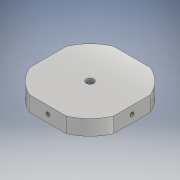
# Autodesk Inventor part: Bottom
Saved by Autodesk Inventor 2017 (Build 210142000, 142)
## iProperties
Created: 2016-06-22
Part Number: Bottom
Material: Generic
Document SubType Name: Modeling
Designer: Andres
Density: 1 g/cm^3
Appearance: Aluminum - Polished
Author: Andres
Autodesk Inventor part; units mm, degrees
ref_plane "YZ Plane" through (0, 0, 0) normal (1, 0, 0) x (0, 1, 0)
ref_plane "XZ Plane" through (0, 0, 0) normal (0, 1, 0) x (-1, 0, 0)
ref_plane "XY Plane" through (0, 0, 0) normal (0, 0, 1) x (1, 0, 0)
sketch "Sketch1" plane through (0, 0, 0) normal (0, 0, 1) x (1, 0, 0)
  circle A0 centre (0, 0) radius 30
  dimension "d0" = 60
  constraints: 1 centre point, 1 coincident
  measures "d0" diameter of A0
extrude "Extrusion1" add sketch "Sketch1" along normal blind 10
sketch "Sketch2" plane through (0, 0, 10) normal (0, 0, 1) x (1, 0, 0)
  line L0 (-27.5, -27.5) -> (27.5, -27.5)
  line L1 (27.5, -27.5) -> (27.5, 27.5)
  line L2 (27.5, 27.5) -> (-27.5, 27.5)
  line L3 (-27.5, 27.5) -> (-27.5, -27.5)
  line L4 (-27.5, -27.5) -> (27.5, 27.5) construction
  line L5 (27.5, -27.5) -> (-27.5, 27.5) construction
  point P0 (0, 0)
  dimension "d3" = 55
  dimension "d4" = 55
  constraints: 12 end point, 2 midpoint, 2 parallel, 1 horizontal, 1 perpendicular
  measures "d3" distance of L2.end L1.end
  measures "d4" distance of L1.end L0.end
extrude "Extrusion2" cut sketch "Sketch2" against normal blind 10 keep common part
sketch "Sketch3" plane through (-27.5, -11.9896, 10) normal (-1, 0, 0) x (0, 0, 1)
  point P0 (-10, 11.9896)
sketch "Sketch4" plane through (0, 0, 10) normal (0, 0, 1) x (1, 0, 0)
  circle A0 centre (0, 0) radius 2.5
  dimension "d7" = 5
  constraints: 1 centre point, 1 coincident
  measures "d7" diameter of A0
extrude "Extrusion3" cut sketch "Sketch4" against normal blind 10
sketch "Sketch9" plane through (-11.9896, -27.5, 10) normal (0, -1, 0) x (1, 0, 0)
  line L0 (23.9792, 0) -> (0, 0) projected
  point P0 (11.9896, -10)
  point P1 (11.9896, -5)
  point P2 (11.9896, 0)
  dimension "d42" = 5
  constraints: 1 midpoint, 1 vertical alignment
  measures "d42" distance from line of L0 point (11.99, -5)
hole "Hole1" at (0, -27.5, 5) direction (0, 1, 0) diameter 2.642 end through all thread size "6-32 UNC" class "3B" standard "ANSI Unified Screw Threads"
pattern_circular "Circular Pattern1" count 2 over 90 about axis through (0, 0, 10) along (0, 0, -1) of "Hole1"
body "Solid1"
